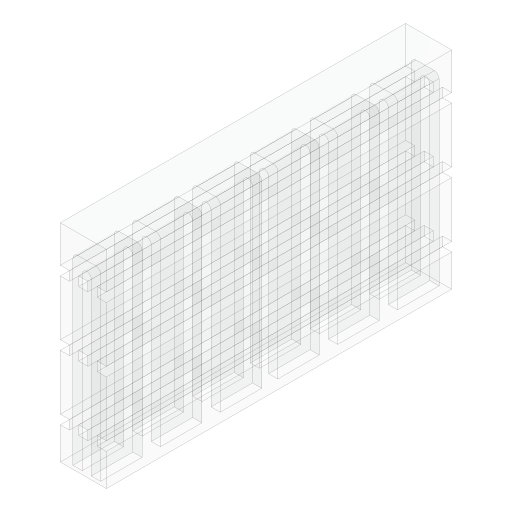
# Autodesk Inventor part: storage
Saved by Autodesk Inventor 2023 (Build 270158000, 158)
## iProperties
Created: 2023-11-13
Part Number: storage
Material: 聚碳酸酯，透明
Document SubType Name: Modeling
Designer: byfbi
Density: 1.2 g/cm^3
Appearance: 聚碳酸酯 - 透明
Author: byfbi
Autodesk Inventor part; units mm, degrees
ref_plane "YZ Plane" through (0, 0, 0) normal (1, 0, 0) x (0, 1, 0)
sketch "草图1" plane through (0, 0, 0) normal (0, 1, 0) x (-1, 0, 0)
  line L0 (50, -375) -> (-50, -375)
  line L1 (-50, -375) -> (-50, 375)
  line L2 (-50, 375) -> (50, 375)
  line L3 (50, 375) -> (50, -375)
  line L4 (50, -375) -> (-50, 375) construction
  line L5 (-50, -375) -> (50, 375) construction
  point P0 (0, 0)
  dimension "d0" = 100
  dimension "d1" = 750
  constraints: 12 end point, 2 midpoint, 2 parallel, 1 horizontal, 1 perpendicular
  measures "d0" distance of L1.end L2.end
  measures "d1" distance of L0.end L1.end
extrude "拉伸1" add sketch "草图1" along normal blind 450
sketch "草图2" plane through (0, 0, 0) normal (0, -1, 0) x (1, 0, 0)
  line L0 (-50, 375) -> (50, 375) projected
  line L1 (-50, -375) -> (-50, 375) projected
  line L2 (50, -375) -> (-50, -375) projected
  line L3 (50, 375) -> (50, -375) projected
  line L4 (30, 367.5) -> (10, 367.5)
  line L5 (10, 367.5) -> (10, 277.5)
  line L6 (10, 277.5) -> (30, 277.5)
  line L7 (30, 277.5) -> (30, 367.5)
  line L8 (30, 367.5) -> (10, 277.5) construction
  line L9 (10, 367.5) -> (30, 277.5) construction
  line L10 (30, 237.5) -> (10, 237.5)
  line L11 (10, 237.5) -> (10, 147.5)
  line L12 (10, 147.5) -> (30, 147.5)
  line L13 (30, 147.5) -> (30, 237.5)
  line L14 (30, 107.5) -> (10, 107.5)
  line L15 (10, 107.5) -> (10, 17.5)
  line L16 (10, 17.5) -> (30, 17.5)
  line L17 (30, 17.5) -> (30, 107.5)
  line L18 (50, 0) -> (-50, 0)
  line L19 (-50, -375) -> (-50, 375) projected
  line L20 (0, 375) -> (0, -375)
  line L21 (30, -367.5) -> (10, -367.5)
  line L22 (10, -367.5) -> (10, -277.5)
  line L23 (10, -277.5) -> (30, -277.5)
  line L24 (30, -277.5) -> (30, -367.5)
  line L25 (30, -367.5) -> (10, -277.5) construction
  line L26 (10, -367.5) -> (30, -277.5) construction
  line L27 (30, -237.5) -> (10, -237.5)
  line L28 (30, -147.5) -> (30, -237.5)
  line L29 (10, -237.5) -> (10, -147.5)
  line L30 (10, -147.5) -> (30, -147.5)
  line L31 (30, -107.5) -> (10, -107.5)
  line L32 (30, -17.5) -> (30, -107.5)
  line L33 (10, -107.5) -> (10, -17.5)
  line L34 (10, -17.5) -> (30, -17.5)
  line L35 (-30, 367.5) -> (-10, 367.5)
  line L36 (-10, 367.5) -> (-10, 277.5)
  line L37 (-10, 277.5) -> (-30, 277.5)
  line L38 (-30, 277.5) -> (-30, 367.5)
  line L39 (-30, 367.5) -> (-10, 277.5) construction
  line L40 (-10, 367.5) -> (-30, 277.5) construction
  line L41 (-30, 237.5) -> (-10, 237.5)
  line L42 (-30, 147.5) -> (-30, 237.5)
  line L43 (-10, 237.5) -> (-10, 147.5)
  line L44 (-10, 147.5) -> (-30, 147.5)
  line L45 (-30, 107.5) -> (-10, 107.5)
  line L46 (-30, 17.5) -> (-30, 107.5)
  line L47 (-10, 107.5) -> (-10, 17.5)
  line L48 (-10, 17.5) -> (-30, 17.5)
  line L49 (-30, -367.5) -> (-10, -367.5)
  line L50 (-10, -147.5) -> (-30, -147.5)
  line L51 (-10, -237.5) -> (-10, -147.5)
  line L52 (-30, -237.5) -> (-10, -237.5)
  line L53 (-30, -147.5) -> (-30, -237.5)
  line L54 (-10, -277.5) -> (-30, -277.5)
  line L55 (-10, -367.5) -> (-10, -277.5)
  line L56 (-30, -277.5) -> (-30, -367.5)
  line L57 (-30, -367.5) -> (-10, -277.5) construction
  line L58 (-10, -367.5) -> (-30, -277.5) construction
  line L59 (-30, -107.5) -> (-10, -107.5)
  line L60 (-30, -17.5) -> (-30, -107.5)
  line L61 (-10, -107.5) -> (-10, -17.5)
  line L62 (-10, -17.5) -> (-30, -17.5)
  point P0 (0, 0)
  point P1 (20, 322.5)
  point P2 (20, 277.5)
  point P3 (20, 237.5)
  point P4 (20, 107.5)
  point P5 (20, 147.5)
  point P6 (20, -322.5)
  point P7 (20, -277.5)
  point P8 (20, -237.5)
  point P9 (20, -107.5)
  point P10 (20, -147.5)
  point P11 (-20, 322.5)
  point P12 (-20, 277.5)
  point P13 (-20, 237.5)
  point P14 (-20, 107.5)
  point P15 (-20, 147.5)
  point P16 (-20, -147.5)
  point P17 (-20, -237.5)
  point P18 (-20, -277.5)
  point P19 (-20, -322.5)
  point P20 (-20, -107.5)
  dimension "d4" = 20
  dimension "d5" = 90
  dimension "d6" = 97.5
  dimension "d7" = 20
  dimension "d8" = 20
  dimension "d9" = 90
  dimension "d10" = 20
  dimension "d11" = 90
  dimension "d12" = 40
  dimension "d13" = 40
  constraints: 116 end point, 51 symmetric about line, 10 midpoint, 6 parallel, 3 horizontal, 3 perpendicular
  measures "d4" distance of L6.end L5.end
  measures "d5" distance of L5.end L4.end
  measures "d6" distance from line of L0 point (20, 277.5)
  measures "d7" distance between parallel lines of L3 L7
  measures "d8" distance of L13.start L11.end
  measures "d9" distance of L11.end L10.end
  measures "d10" distance of L17.start L15.end
  measures "d11" distance of L15.end L14.end
  measures "d12" distance of point (20, 237.5) point (20, 277.5)
  measures "d13" distance of point (20, 107.5) point (20, 147.5)
extrude "拉伸2" cut sketch "草图2" against normal blind 400 contours L7 L6 L5 L4 | L13 L12 L11 L10 | L17 L16 L15 L14 | L21 L22 L23 L24 | L27 L29 L30 L28 | L31 L33 L34 L32 | L35 L36 L37 L38 | L41 L43 L44 L42 | L45 L47 L48 L46 | L56 L54 L55 L49 | L51 L52 L53 L50 | L60 L62 L61 L59
ref_plane "工作平面1" through (20, 0, 375) normal (1, 0, 0) x (0, 0, -1)
sketch "草图3" plane through (20, 0, 375) normal (1, 0, 0) x (0, 0, -1)
  line L0 (7.5, 0) -> (97.5, 0) projected
  line L1 (7.5, 0) -> (7.5, 400) projected
  line L2 (7.5, 400) -> (97.5, 400) projected
  line L3 (97.5, 0) -> (97.5, 400) projected
  line L4 (137.5, 0) -> (227.5, 0) projected
  line L5 (137.5, 0) -> (137.5, 400) projected
  line L6 (137.5, 400) -> (227.5, 400) projected
  line L7 (227.5, 0) -> (227.5, 400) projected
  line L8 (267.5, 0) -> (357.5, 0) projected
  line L9 (267.5, 0) -> (267.5, 400) projected
  line L10 (267.5, 400) -> (357.5, 400) projected
  line L11 (357.5, 0) -> (357.5, 400) projected
  line L12 (392.5, 0) -> (482.5, 0) projected
  line L13 (392.5, 0) -> (392.5, 400) projected
  line L14 (392.5, 400) -> (482.5, 400) projected
  line L15 (482.5, 0) -> (482.5, 400) projected
  line L16 (522.5, 0) -> (612.5, 0) projected
  line L17 (522.5, 0) -> (522.5, 400) projected
  line L18 (522.5, 400) -> (612.5, 400) projected
  line L19 (612.5, 0) -> (612.5, 400) projected
  line L20 (652.5, 0) -> (742.5, 0) projected
  line L21 (652.5, 0) -> (652.5, 400) projected
  line L22 (652.5, 400) -> (742.5, 400) projected
  line L23 (742.5, 0) -> (742.5, 400) projected
  line L24 (7.5, 0) -> (7.5, 400) projected
  line L25 (7.5, 400) -> (57.5, 400)
  line L26 (57.5, 400) -> (57.5, 390)
  line L27 (57.5, 390) -> (7.5, 390)
  line L28 (7.5, 390) -> (7.5, 400)
  line L29 (227.5, 400) -> (137.5, 400) projected
  line L30 (137.5, 400) -> (187.5, 400)
  line L31 (187.5, 400) -> (187.5, 390)
  line L32 (187.5, 390) -> (137.5, 390)
  line L33 (137.5, 390) -> (137.5, 400)
  line L34 (267.5, 0) -> (267.5, 400) projected
  line L35 (267.5, 400) -> (317.5, 400)
  line L36 (317.5, 400) -> (317.5, 390)
  line L37 (317.5, 390) -> (267.5, 390)
  line L38 (267.5, 390) -> (267.5, 400)
  line L39 (482.5, 400) -> (392.5, 400) projected
  line L40 (392.5, 400) -> (442.5, 400)
  line L41 (442.5, 400) -> (442.5, 390)
  line L42 (442.5, 390) -> (392.5, 390)
  line L43 (392.5, 390) -> (392.5, 400)
  line L44 (612.5, 400) -> (522.5, 400) projected
  line L45 (522.5, 400) -> (572.5, 400)
  line L46 (572.5, 400) -> (572.5, 390)
  line L47 (572.5, 390) -> (522.5, 390)
  line L48 (522.5, 390) -> (522.5, 400)
  line L49 (652.5, 400) -> (702.5, 400)
  line L50 (702.5, 400) -> (702.5, 390)
  line L51 (702.5, 390) -> (652.5, 390)
  line L52 (652.5, 390) -> (652.5, 400)
  point P0 (375, 0)
  point P1 (712.5, 390)
  point P2 (587.5, 390)
  point P3 (462.5, 390)
  point P4 (267.5, 390)
  point P5 (337.5, 390)
  point P6 (137.5, 390)
  point P7 (212.5, 390)
  point P8 (87.5, 390)
  dimension "d17" = 50
  dimension "d18" = 10
  dimension "d19" = 50
  dimension "d20" = 10
  dimension "d21" = 50
  dimension "d22" = 10
  dimension "d23" = 50
  dimension "d24" = 10
  dimension "d25" = 50
  dimension "d26" = 10
  dimension "d27" = 50
  dimension "d28" = 10
  constraints: 48 end point, 12 parallel, 6 horizontal, 6 perpendicular
  measures "d17" distance of L26.end L27.end
  measures "d18" distance of L25.end L26.end
  measures "d19" distance of L31.end L32.end
  measures "d20" distance of L30.end L31.end
  measures "d21" distance of L36.end L37.end
  measures "d22" distance of L35.end L36.end
  measures "d23" distance of L41.end L42.end
  measures "d24" distance of L40.end L41.end
  measures "d25" distance of L46.end L47.end
  measures "d26" distance of L45.end L46.end
  measures "d27" distance of L50.end L51.end
  measures "d28" distance of L49.end L50.end
extrude "拉伸3" [suppressed]
fillet "圆角1" [suppressed]
fillet "圆角2" [suppressed]
ref_plane "工作平面2" through (-10, 0, -375) normal (-1, 0, 0) x (0, 0, 1)
sketch "草图4" plane through (-10, 0, -375) normal (-1, 0, 0) x (0, 0, 1)
  line L0 (7.5, 0) -> (97.5, 0) projected
  line L1 (7.5, 0) -> (7.5, 400) projected
  line L2 (7.5, 400) -> (97.5, 400) projected
  line L3 (97.5, 0) -> (97.5, 400) projected
  line L4 (137.5, 0) -> (227.5, 0) projected
  line L5 (137.5, 0) -> (137.5, 400) projected
  line L6 (137.5, 400) -> (227.5, 400) projected
  line L7 (227.5, 0) -> (227.5, 400) projected
  line L8 (267.5, 0) -> (357.5, 0) projected
  line L9 (267.5, 0) -> (267.5, 400) projected
  line L10 (267.5, 400) -> (357.5, 400) projected
  line L11 (357.5, 0) -> (357.5, 400) projected
  line L12 (392.5, 0) -> (482.5, 0) projected
  line L13 (392.5, 0) -> (392.5, 400) projected
  line L14 (392.5, 400) -> (482.5, 400) projected
  line L15 (482.5, 0) -> (482.5, 400) projected
  line L16 (522.5, 0) -> (612.5, 0) projected
  line L17 (522.5, 0) -> (522.5, 400) projected
  line L18 (522.5, 400) -> (612.5, 400) projected
  line L19 (612.5, 0) -> (612.5, 400) projected
  line L20 (652.5, 0) -> (742.5, 0) projected
  line L21 (652.5, 0) -> (652.5, 400) projected
  line L22 (652.5, 400) -> (742.5, 400) projected
  line L23 (742.5, 0) -> (742.5, 400) projected
  line L24 (7.5, 400) -> (97.5, 400)
  line L25 (97.5, 400) -> (97.5, 380)
  line L26 (97.5, 380) -> (7.5, 380)
  line L27 (7.5, 380) -> (7.5, 400)
  line L28 (137.5, 400) -> (227.5, 400)
  line L29 (227.5, 400) -> (227.5, 380)
  line L30 (227.5, 380) -> (137.5, 380)
  line L31 (137.5, 380) -> (137.5, 400)
  line L32 (267.5, 400) -> (357.5, 400)
  line L33 (357.5, 400) -> (357.5, 380)
  line L34 (357.5, 380) -> (267.5, 380)
  line L35 (267.5, 380) -> (267.5, 400)
  line L36 (392.5, 400) -> (482.5, 400)
  line L37 (482.5, 400) -> (482.5, 380)
  line L38 (482.5, 380) -> (392.5, 380)
  line L39 (392.5, 380) -> (392.5, 400)
  line L40 (522.5, 400) -> (612.5, 400)
  line L41 (612.5, 400) -> (612.5, 380)
  line L42 (612.5, 380) -> (522.5, 380)
  line L43 (522.5, 380) -> (522.5, 400)
  line L44 (652.5, 400) -> (742.5, 400)
  line L45 (742.5, 400) -> (742.5, 380)
  line L46 (742.5, 380) -> (652.5, 380)
  line L47 (652.5, 380) -> (652.5, 400)
  point P0 (375, 0)
  dimension "d34" = 90
  dimension "d35" = 20
  dimension "d36" = 90
  dimension "d37" = 20
  dimension "d38" = 90
  dimension "d39" = 20
  dimension "d40" = 90
  dimension "d41" = 20
  dimension "d42" = 90
  dimension "d43" = 20
  dimension "d44" = 90
  dimension "d45" = 20
  constraints: 48 end point, 12 parallel, 6 horizontal, 6 perpendicular
  measures "d34" distance of L25.end L26.end
  measures "d35" distance of L24.end L25.end
  measures "d36" distance of L29.end L30.end
  measures "d37" distance of L28.end L29.end
  measures "d38" distance of L33.end L34.end
  measures "d39" distance of L32.end L33.end
  measures "d40" distance of L37.end L38.end
  measures "d41" distance of L36.end L37.end
  measures "d42" distance of L41.end L42.end
  measures "d43" distance of L40.end L41.end
  measures "d44" distance of L45.end L46.end
  measures "d45" distance of L44.end L45.end
extrude "拉伸4" cut sketch "草图4" against normal blind 20 contours L1 L2 L3 L26 | L5 L6 L7 L30 | L9 L10 L11 L34 | L13 L14 L15 L38 | L17 L18 L19 L42 | L21 L22 L23 L46
fillet "圆角3" radius 10 24 edges at (30, 400, -322.5) (-30, 400, -322.5) (10, 380, -322.5) (-10, 380, -322.5) (30, 400, -192.5) (-30, 400, -192.5) (10, 380, -192.5) (-10, 380, -192.5) (-10, 380, 62.5) (10, 380, 62.5) (-30, 400, -62.5) (30, 400, -62.5) (30, 400, 62.5) (-30, 400, 62.5) (10, 380, 192.5) (-10, 380, 192.5) (30, 400, 192.5) (-30, 400, 192.5) (10, 380, 322.5) (-10, 380, 322.5) (30, 400, 322.5) (-30, 400, 322.5) (-10, 380, -62.5) (10, 380, -62.5)
sketch "草图5" plane through (50, 0, -375) normal (0, 0, -1) x (-1, 0, 0)
  arc A0 (60, 370) -> (40, 370) centre (50, 370) ccw projected
  line L0 (40, 0) -> (40, 370) projected
  line L1 (60, 0) -> (60, 370) projected
  arc A1 (30, 400) -> (20, 390) centre (30, 390) ccw projected
  line L2 (30, 400) -> (70, 400) projected
  arc A2 (80, 390) -> (70, 400) centre (70, 390) ccw projected
  line L3 (20, 0) -> (20, 390) projected
  line L4 (80, 0) -> (80, 390) projected
  line L5 (0, 0) -> (0, 450) projected
  line L6 (100, 0) -> (100, 450) projected
  line L7 (40, 0) -> (40, 370) projected
  line L8 (40, 370) -> (60, 370)
  line L9 (60, 370) -> (60, 350)
  line L10 (60, 350) -> (40, 350)
  line L11 (40, 350) -> (40, 370)
  line L12 (40, 230) -> (60, 230)
  line L13 (60, 230) -> (60, 210)
  line L14 (60, 210) -> (40, 210)
  line L15 (40, 210) -> (40, 230)
  line L16 (40, 90) -> (60, 90)
  line L17 (60, 90) -> (60, 70)
  line L18 (60, 70) -> (40, 70)
  line L19 (40, 70) -> (40, 90)
  line L20 (0, 370) -> (20, 370)
  line L21 (20, 370) -> (20, 350)
  line L22 (20, 350) -> (0, 350)
  line L23 (0, 350) -> (0, 370)
  line L24 (80, 0) -> (80, 390) projected
  line L25 (80, 370) -> (100, 370)
  line L26 (100, 370) -> (100, 350)
  line L27 (100, 350) -> (80, 350)
  line L28 (80, 350) -> (80, 370)
  line L29 (0, 230) -> (20, 230)
  line L30 (20, 230) -> (20, 210)
  line L31 (20, 210) -> (0, 210)
  line L32 (0, 210) -> (0, 230)
  line L33 (80, 230) -> (100, 230)
  line L34 (100, 230) -> (100, 210)
  line L35 (100, 210) -> (80, 210)
  line L36 (80, 210) -> (80, 230)
  line L37 (0, 0) -> (0, 450) projected
  line L38 (0, 90) -> (20, 90)
  line L39 (20, 90) -> (20, 70)
  line L40 (20, 70) -> (0, 70)
  line L41 (0, 70) -> (0, 90)
  line L42 (80, 90) -> (100, 90)
  line L43 (100, 90) -> (100, 70)
  line L44 (100, 70) -> (80, 70)
  line L45 (80, 70) -> (80, 90)
  point P0 (50, 0)
  point P1 (50, 230)
  point P2 (50, 350)
  point P3 (50, 90)
  point P4 (50, 210)
  dimension "d49" = 20
  dimension "d50" = 20
  dimension "d51" = 20
  dimension "d52" = 20
  dimension "d53" = 20
  dimension "d54" = 20
  dimension "d55" = 120
  dimension "d56" = 120
  dimension "d57" = 20
  dimension "d58" = 20
  dimension "d59" = 20
  dimension "d60" = 20
  dimension "d61" = 20
  dimension "d62" = 20
  dimension "d63" = 20
  dimension "d64" = 20
  dimension "d65" = 20
  dimension "d66" = 20
  dimension "d67" = 20
  dimension "d68" = 20
  constraints: 72 end point, 18 parallel, 11 point on line, 9 horizontal, 9 perpendicular, 4 midpoint
  measures "d49" distance of L9.end L10.end
  measures "d50" distance of L8.end L9.end
  measures "d51" distance of L13.end L14.end
  measures "d52" distance of L12.end L13.end
  measures "d53" distance of L17.end L18.end
  measures "d54" distance of L16.end L17.end
  measures "d55" distance of point (50, 230) point (50, 350)
  measures "d56" distance of point (50, 90) point (50, 210)
  measures "d57" distance of L21.end L22.end
  measures "d58" distance of L20.end L21.end
  measures "d59" distance of L26.end L27.end
  measures "d60" distance of L25.end L26.end
  measures "d61" distance of L30.end L31.end
  measures "d62" distance of L29.end L30.end
  measures "d63" distance of L34.end L35.end
  measures "d64" distance of L33.end L34.end
  measures "d65" distance of L39.end L40.end
  measures "d66" distance of L38.end L39.end
  measures "d67" distance of L43.end L44.end
  measures "d68" distance of L42.end L43.end
extrude "拉伸5" cut sketch "草图5" against normal blind 750 contours L1 L10 L0 L8 | L1 L14 L0 L12 | L1 L18 L0 L16 | L3 L22 L5 L20 | L25 L6 L27 L4 | L3 L31 L5 L29 | L33 L6 L35 L4 | L3 L40 L5 L38 | L42 L6 L44 L4
